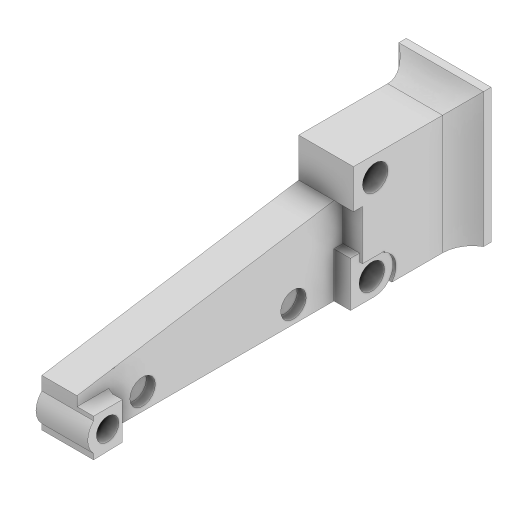
# Autodesk Inventor part: MotorAP
Saved by Autodesk Inventor 2023 (Build 270158030, 158C)
## iProperties
Created: 2022-08-10
Part Number: MotorAP
Material: Generic
Document SubType Name: Modeling
Designer: Ben
Density: 1 g/cm^3
Appearance: Default
Author: Ben
Autodesk Inventor part; units mm, degrees
sketch "Sketch1" plane through (0, 0, 0) normal (0, 0, 1) x (1, 0, 0)
  line L0 (0, 28.725) -> (20.5901, 28.725) projected
  line L1 (8.1353, 17.1738) -> (8.1353, 20.6738) projected
  line L2 (4.6353, 17.1738) -> (8.1353, 17.1738) projected
  line L3 (4.6353, 20.6738) -> (4.6353, 17.1738) projected
  line L4 (8.1353, 20.6738) -> (4.6353, 20.6738) projected
  line L5 (15.9861, 17.1738) -> (15.9861, 20.6738) projected
  line L6 (12.4861, 17.1738) -> (15.9861, 17.1738) projected
  line L7 (12.4861, 20.6738) -> (12.4861, 17.1738) projected
  line L8 (15.9861, 20.6738) -> (12.4861, 20.6738) projected
  circle A0 centre (14.2361, 18.9238) radius 1.75
  line L9 (0, 28.725) -> (0, 14.1337) projected
  line L10 (20.5901, 14.1337) -> (20.5901, 28.725) projected
  line L11 (0, 14.1337) -> (20.5901, 14.1337) projected
  constraints: 1 centre point, 1 tangent
sketch "Sketch2" plane through (0, 0, 0) normal (0, 0, 1) x (1, 0, 0)
  line L0 (13.8808, 28.6928) -> (10.5387, 28.6928)
  line L1 (10.5387, 28.6928) -> (10.5387, 20.7516)
  line L2 (10.5387, 20.7516) -> (13.8808, 20.7516)
  line L3 (14.1861, 26.5937) -> (14.1861, 28.0937)
  line L4 (14.1861, 20.7516) -> (13.8808, 20.7516)
  line L5 (13.8808, 28.6928) -> (14.1861, 28.6928)
  line L6 (14.5861, 22.7938) -> (13.9861, 22.7938)
  line L7 (14.1861, 26.0937) -> (14.5861, 26.0937)
  line L8 (14.1861, 26.0937) -> (15.1861, 26.0937)
  line L9 (15.1861, 26.0937) -> (15.1861, 22.7938)
  line L10 (15.1861, 22.7938) -> (14.1861, 22.7938)
  line L11 (14.1861, 28.6928) -> (14.1861, 26.0937)
  line L12 (14.1861, 22.7938) -> (14.1861, 20.7516)
  point P0 (0, 0)
  dimension "d2" = 1
  constraints: 26 end point, 4 perpendicular, 3 horizontal, 3 vertical, 2 parallel, 2 point on line, 6 other
  measures "d2" distance of L7.start L8.end
ref_plane "Work Plane1" through (12.8861, 20.2938, 3.59) normal (0, 0, -1) x (0, 1, 0)
extrude "Extrusion1" add sketch "Sketch2" along normal up to surface (3.59 mm away)
sketch "Sketch3" plane through (10.5387, 20.7516, 0) normal (-1, 0, 0) x (0, 0, 1)
  circle A0 centre (2.14, 6.5922) radius 0.75 projected
  circle A1 centre (2.17, 0.7922) radius 0.75 projected
  circle A2 centre (2.14, 6.5922) radius 0.85
  circle A3 centre (2.17, 0.7922) radius 0.85
  point P0 (0, -20.7516)
  dimension "d48" = 1.7
  dimension "d49" = 1.7
  constraints: 2 centre point, 2 coincident
  measures "d48" diameter of A2
  measures "d49" diameter of A3
extrude "Extrusion2" cut sketch "Sketch3" against normal up to next contours A0 | A1
ref_plane "Work Plane2" through (13.9861, 21.5438, 19.605) normal (-1, 0, 0) x (0, -1, 0)
sketch "Sketch5" plane through (13.9861, 21.5438, 19.605) normal (-1, 0, 0) x (0, -1, 0)
  line L0 (-4.5499, -16.015) -> (-7.149, -16.015) projected
  line L1 (-7.149, -16.015) -> (0.7922, -16.015) projected
  line L2 (0.7922, -16.015) -> (-1.25, -16.015) projected
  line L3 (-1.25, -16.015) -> (-4.5499, -16.015) projected
  circle A0 centre (0, 0.165) radius 0.75 projected
  line L4 (-4.5499, -16.015) -> (-7.149, -16.015) projected
  line L5 (1.3262, 1.5964) -> (-7.149, 1.5964)
  line L6 (-7.149, 1.5964) -> (-7.149, -16.015)
  line L7 (-7.149, -16.015) -> (1.3262, -16.015)
  line L8 (-4.5499, -19.605) -> (-4.5499, -16.015) projected
  line L9 (-1.7621, 1.5964) -> (-4.5499, -16.015)
  line L10 (0.7922, -19.605) -> (0.7922, -16.015) projected
  line L11 (0.7922, -19.605) -> (0.7922, -16.015) projected
  line L12 (0.7922, -16.015) -> (-1.25, -16.015) projected
  line L13 (0.7922, -16.015) -> (1.3262, 1.5964)
  circle A1 centre (0, 0.165) radius 0.85
  point P0 (21.5438, -19.605)
  dimension "d47" = 1.7
  constraints: 10 end point, 1 centre point, 1 coincident, 1 horizontal, 1 parallel, 1 perpendicular, 1 point on line
  measures "d47" diameter of A1
extrude "Extrusion3" add sketch "Sketch5" along normal up to surface (3.4474 mm away) contours L9 L5 L13 L1
sketch "Sketch6" plane through (13.9861, 21.5438, 19.605) normal (1, 0, 0) x (0, 0, -1)
  line L0 (16.015, 4.5499) -> (16.015, 7.149) projected
  line L1 (16.015, -0.7922) -> (-1.5964, -1.3262) projected
  line L2 (16.015, 7.149) -> (-1.5964, 7.149)
  line L3 (-1.5964, 7.149) -> (-1.5964, -1.3262)
  line L4 (-1.5964, -1.3262) -> (16.015, -1.3262)
  line L5 (16.015, -1.3262) -> (16.015, 7.149)
  point P0 (19.605, -21.5438)
  constraints: 8 end point, 2 parallel, 1 horizontal, 1 perpendicular
ref_plane "Work Plane3" through (12.8861, 20.2938, 3.59) normal (-1, 0, 0) x (0, 0, 1)
extrude "Extrusion4" cut sketch "Sketch6" against normal up to surface (1.1 mm away) contours L5 L1 L3 L2 L0
sketch "Sketch7" plane through (12.8861, 20.7516, 3.59) normal (1, 0, 0) x (0, 0, -1)
  line L0 (-14.6, 7.4422) -> (-14.6, -0.4578) projected
  line L1 (-17.6114, 2.5543) -> (0, 5.3422) projected
  line L2 (-14.6, -0.4578) -> (-14.6, 3.031)
  circle A0 centre (-16.18, 0.7922) radius 0.75 projected
  line L3 (0, 0) -> (-17.6114, -0.5339) projected
  line L4 (-17.6114, -0.5339) -> (-17.6114, 2.5543) projected
  point P0 (3.59, -20.7516)
  point P1 (-14.6, -0.4426)
  constraints: 2 end point, 2 point on line
ref_plane "Work Plane4" through (13.9861, 20.2938, 18.19) normal (-1, 0, 0) x (0, 0, 1)
extrude "Extrusion5" add sketch "Sketch7" along normal up to surface (1.1 mm away)
sketch "Sketch8" plane through (13.9861, 20.3089, 18.19) normal (1, 0, 0) x (0, 0, -1)
  arc A0 (-1.58, 2.4849) -> (-1.58, -0.0151) centre (-1.58, 1.2349) ccw projected
  line L0 (0, 2.5649) -> (-6.5, 2.5649)
  line L1 (-3.0114, -0.0913) -> (0, 0) projected
  line L2 (-3.0114, 2.997) -> (-3.0114, -0.0913) projected
  line L3 (-1.58, 2.4849) -> (-1.58, 2.5649)
  line L4 (-1.58, -0.0151) -> (-1.58, -0.0479)
  circle A1 centre (-1.58, 1.2349) radius 1.325
  line L5 (-2.5138, 2.1749) -> (-2.5138, 2.5649)
  line L6 (-2.5138, 0.2949) -> (-2.5138, -0.0762)
  point P0 (18.19, -20.3089)
  point P1 (-3.0114, 2.5649)
  dimension "d42" = 2.65
  constraints: 10 end point, 6 point on line, 2 point on circle, 1 centre point, 1 coincident, 1 horizontal, 1 perpendicular, 1 vertical, 2 other
  measures "d42" diameter of A1
ref_plane "Work Plane5" through (14.5861, 20.2938, 17.09) normal (1, 0, 0) x (0, 1, 0)
extrude "Extrusion6" add sketch "Sketch8" along normal up to surface (0.6 mm away) contours A1 L6 L1 L2 L0 L5
sketch "Sketch9" plane through (14.1861, 20.7516, 0) normal (1, 0, 0) x (0, 0, -1)
  circle A0 centre (-2.14, 6.5922) radius 0.75 projected
  line L0 (-3.59, 5.3422) -> (-3.59, 7.9412) projected
  line L1 (0, 5.3422) -> (-3.59, 5.3422) projected
  line L2 (0, 5.3422) -> (0, 7.9412) projected
  line L3 (0, 7.9412) -> (-3.59, 7.9412) projected
  line L4 (-3.59, 2.0422) -> (-3.59, 5.3422) projected
  line L5 (0, 2.0422) -> (-3.59, 2.0422) projected
  line L6 (0, 2.0422) -> (0, 5.3422) projected
  line L7 (0, 5.3422) -> (-3.59, 5.3422) projected
  circle A1 centre (-2.17, 0.7922) radius 0.75 projected
  line L8 (-3.59, 0) -> (-3.59, 2.0422) projected
  line L9 (0, 0) -> (-3.59, 0) projected
  line L10 (0, 0) -> (0, 2.0422) projected
  line L11 (0, 2.0422) -> (-3.59, 2.0422) projected
  point P0 (0, -20.7516)
ref_plane "Work Plane6" through (13.9861, 20.2938, 0.75) normal (-1, 0, 0) x (0, 0, 1)
sketch "Sketch10" plane through (14.1861, 20.7516, 0) normal (1, 0, 0) x (0, 0, -1)
  circle A0 centre (-2.17, 0.7922) radius 0.75 projected
  line L0 (-3.59, 0) -> (-3.59, 2.0422) projected
  line L1 (0, 0) -> (-3.59, 0) projected
  line L2 (0, 0) -> (0, 2.0422) projected
  line L3 (0, 2.0422) -> (-3.59, 2.0422) projected
  point P0 (0, -20.7516)
ref_plane "Work Plane7" through (13.9861, 20.2938, 0.75) normal (-1, 0, 0) x (0, 0, 1)
extrude "Extrusion8" cut sketch "Sketch10" against normal up to surface (0.2 mm away)
sketch "Sketch11" plane through (10.5387, 20.2176, 21.2014) normal (0, 0, 1) x (1, 0, 0)
  circle A0 centre (4.4974, 4.8062) radius 2.2 projected
  circle A1 centre (4.4974, 4.8062) radius 2.5
  point P0 (-10.5387, -20.2176)
  dimension "d46" = 5
  constraints: 1 centre point, 1 coincident
  measures "d46" diameter of A1
ref_plane "Work Plane8" through (12.8861, 20.2938, 18.19) normal (0, 0, 1) x (1, 0, 0)
extrude "Extrusion9" cut sketch "Sketch11" against normal up to surface (3.0114 mm away) contours A0 | A1
sketch "Sketch12" plane through (12.8861, 20.7516, 3.59) normal (1, 0, 0) x (0, 0, -1)
  circle A0 centre (-12.75, 0.6922) radius 0.85
  circle A1 centre (-2.7, 0.6922) radius 0.85
  line L0 (-3.4464, 0) -> (-2.0459, 0)
  point P0 (3.59, -20.7516)
  point P1 (-3.1933, 0)
  point P2 (-2.2067, 0)
  dimension "d40" = 1.7
  dimension "d41" = 1.7
  constraints: 2 centre point, 2 end point, 1 horizontal
  measures "d40" diameter of A0
  measures "d41" diameter of A1
extrude "Extrusion10" cut sketch "Sketch12" against normal blind 0.6 contours A0 | A1 L0 picked at (-2.6162, 0.9299)
sketch "Sketch13" plane through (14.1861, 26.0937, 0) normal (1, 0, 0) x (0, 0, -1)
  arc A0 (-2.14, 0) -> (-3.0564, 2.1001) centre (-2.14, 1.25) ccw projected
  line L0 (-1.9353, 2.4831) -> (-1.9353, 2.5991)
  line L1 (0, 2.5991) -> (-3.59, 2.5991) projected
  line L2 (0, 0) -> (0, 2.5991)
  line L3 (-1.6782, 0.0884) -> (-1.6782, 0)
  arc A1 (-2.14, 0) -> (-3.0564, 2.1001) centre (-2.14, 1.25) ccw projected
  circle A2 centre (-2.14, 1.25) radius 1.25
  line L4 (0, 0) -> (-3.59, 0) projected
  line L5 (-1.6782, 0) -> (0, 0)
  point P0 (0, -26.0937)
  constraints: 8 end point, 3 vertical, 2 point on circle, 1 centre point, 1 coincident, 1 concentric, 1 horizontal, 1 point on line
extrude "Extrusion11" add sketch "Sketch13" along normal up to surface (1 mm away) contours A0 L0 L1 L2 L4 L3
sketch "Sketch16" plane through (13.9861, 20.7516, 3.59) normal (1, 0, 0) x (0, 0, -1)
  line L0 (3.59, 7.9412) -> (3.59, 0) projected
  line L1 (3.59, 2.0422) -> (0, 2.0422) projected
  line L2 (3.59, 0) -> (2.0582, 0)
  line L3 (2.0582, 0) -> (2.0582, 2.0422)
  line L4 (2.0582, 2.0422) -> (3.59, 2.0422)
  line L5 (3.59, 2.0422) -> (3.59, 0)
  arc A0 (1.59, -0.4578) -> (1.59, 2.0422) centre (1.59, 0.7922) ccw projected
  point P0 (3.59, -20.7516)
  point P1 (2.0582, 1.9512)
  point P2 (2.5569, 0)
  constraints: 8 end point, 2 parallel, 1 horizontal, 1 perpendicular, 1 point on line
extrude "Extrusion12" add sketch "Sketch16" along normal up to surface (1.2 mm away) contours L0 L2 A0 L3 L1
sketch "Sketch18" plane through (10.5387, 20.2176, 21.2014) normal (-1, 0, 0) x (0, 0, 1)
  arc A0 (-18.3114, 7.1261) -> (-18.3114, 7.1261) centre (-19.0614, 7.1261) ccw projected
  arc A1 (-18.2814, 1.3262) -> (-18.2814, 1.3262) centre (-19.0314, 1.3262) ccw projected
  circle A2 centre (-19.0614, 7.1261) radius 1.25
  circle A3 centre (-19.0314, 1.3262) radius 1.25
  line L0 (-17.6114, 8.4752) -> (-17.6114, 5.8761) projected
  line L1 (-17.6114, 8.4752) -> (-17.6114, 0.5362)
  line L2 (-20.1683, 0.5339) -> (-17.6114, 0.5339) projected
  line L3 (-17.6114, 0.5362) -> (-17.6114, 0.5339)
  line L4 (-20.6002, 0.5339) -> (-20.6002, 8.4752) projected
  line L5 (-17.6114, 8.4752) -> (-20.6002, 8.4752)
  line L6 (-20.6002, 8.4752) -> (-20.6002, 0.5339)
  line L7 (-20.6002, 0.5339) -> (-19.9983, 0.5339)
  line L8 (-20.6002, 0.5339) -> (-17.6114, 0.5339)
  point P0 (-21.2014, -20.2176)
  point P1 (-18.0645, 0.5339)
  dimension "d27" = 2.5
  constraints: 12 end point, 3 perpendicular, 2 coincident, 1 centre point, 1 collinear, 1 point on line, 1 vertical, 3 other
extrude "Extrusion14" cut sketch "Sketch18" along normal through all contours A0 | A1 | A2 | A3 L2 picked at (-17.9599, 1.4249)
sketch "Sketch19" plane through (15.1861, 22.7938, 3.59) normal (1, 0, 0) x (0, 0, -1)
  line L0 (1.9118, 3.2999) -> (0, 3.2999) projected
  line L1 (2.9889, -2.0422) -> (2.9889, 5.899) projected
  line L2 (1.0967, 3.2999) -> (2.9889, 3.2999)
  line L3 (2.9889, 3.2999) -> (2.9889, 5.899)
  line L4 (2.9889, 5.899) -> (1.0967, 5.899)
  line L5 (1.0967, 5.899) -> (1.0967, 3.2999)
  circle A0 centre (1.4413, 4.5476) radius 1.5803
  point P0 (3.59, -22.7938)
  point P1 (0.4713, 3.2999)
  point P2 (2.4113, 3.2999)
  constraints: 8 end point, 2 parallel, 1 centre point, 1 horizontal, 1 perpendicular, 1 point on line
ref_plane "Work Plane9" through (14.5861, 26.0937, 0.89) normal (1, 0, 0) x (0, 1, 0)
extrude "Extrusion15" cut sketch "Sketch19" against normal up to surface (0.6 mm away) contours L2 A0 L0 | L0 L5 L4 A0 L1 L2 | A0 L1 L2 | L4 L1 A0
sketch "Sketch20" plane through (15.1861, 22.7938, 3.59) normal (1, 0, 0) x (0, 0, -1)
  line L0 (2.0582, 0) -> (0, 0) projected
  line L1 (2.9889, -2.0422) -> (3.59, -2.0422) projected
  line L2 (2.0582, 0) -> (2.9889, 0)
  line L3 (2.9889, 0) -> (2.9889, -2.0422)
  line L4 (2.9889, -2.0422) -> (2.0582, -2.0422)
  line L5 (2.0582, -2.0422) -> (2.0582, 0)
  circle A0 centre (1.4197, -1.2443) radius 1.5589
  point P0 (3.59, -22.7938)
  point P1 (2.3588, 0)
  point P2 (0.4807, 0)
  constraints: 8 end point, 2 parallel, 1 centre point, 1 horizontal, 1 perpendicular
ref_plane "Work Plane10" through (14.5861, 20.2938, 0.75) normal (1, 0, 0) x (0, 1, 0)
extrude "Extrusion16" cut sketch "Sketch20" against normal up to surface (0.6 mm away) contours L0 A0 L2 | L2 A0 L4 L5 | L2 L3 L4 A0
sketch "Sketch21" plane through (15.1861, 22.7938, 3.59) normal (1, 0, 0) x (0, 0, -1)
  line L0 (0.4713, 3.2999) -> (1.9118, 3.2999) projected
  arc A0 (0.4713, 3.2999) -> (2.4113, 3.2999) centre (1.4413, 4.5476) ccw projected
  line L1 (2.9889, 3.2999) -> (2.4113, 3.2999) projected
  line L2 (2.9889, 5.899) -> (2.9889, 3.2999) projected
  line L3 (1.6547, 5.899) -> (2.9889, 5.899) projected
  line L4 (1.6547, 5.783) -> (1.6547, 5.899) projected
  arc A1 (1.9118, 3.3884) -> (1.6547, 5.783) centre (1.45, 4.5499) ccw projected
  line L5 (1.9118, 3.2999) -> (1.9118, 3.3884) projected
  arc A2 (2.3588, 0) -> (0.4807, 0) centre (1.4197, -1.2443) ccw projected
  line L6 (2.3588, 0) -> (2.9889, 0) projected
  line L7 (2.9889, 3.2999) -> (2.4113, 3.2999) projected
  arc A3 (0.4713, 3.2999) -> (2.4113, 3.2999) centre (1.4413, 4.5476) ccw projected
  line L8 (0.4713, 3.2999) -> (0, 3.2999) projected
  line L9 (0, 0) -> (0, 3.2999) projected
  line L10 (0.4807, 0) -> (0, 0) projected
  line L11 (0, 0) -> (0, 3.2999) projected
  line L12 (0.4713, 3.2999) -> (1.9118, 3.2999) projected
  line L13 (0, 0.5118) -> (0.6, 0.5118)
  line L14 (0.6, 0.5118) -> (0.6, 3.2999)
  line L15 (0.6, 3.2999) -> (0, 3.2999)
  line L16 (0, 3.2999) -> (0, 0.5118)
  line L17 (2.9889, 0) -> (2.9889, -2.0422) projected
  line L18 (3.59, -2.0422) -> (2.9889, -2.0422) projected
  line L19 (3.59, 5.899) -> (3.59, -2.0422) projected
  line L20 (2.9889, 5.899) -> (3.59, 5.899) projected
  line L21 (2.9889, 5.899) -> (2.9889, 3.2999) projected
  point P0 (3.59, -22.7938)
  point P1 (0.6, 3.2098)
  point P2 (0.4713, 3.2999)
  dimension "d34" = 0.6
  constraints: 8 end point, 2 parallel, 2 point on line, 1 horizontal, 1 perpendicular
  measures "d34" distance of L15.end L14.end
extrude "Extrusion17" cut sketch "Sketch21" against normal up to surface (2.3 mm away) contours L0 L14 A0 | A0 L14 L13 L9 L8
sketch "Sketch22" plane through (13.9861, 20.7516, 3.59) normal (1, 0, 0) x (0, 0, -1)
  line L0 (2.0582, 1.9512) -> (2.0582, 2.0422) projected
  line L1 (2.0582, 2.0422) -> (0, 2.0422) projected
  line L2 (0, 0) -> (0, 2.0422) projected
  line L3 (2.5569, 0) -> (0, 0) projected
  arc A0 (2.5569, 0) -> (2.0582, 1.9512) centre (1.59, 0.7922) ccw projected
  circle A1 centre (1.42, 0.7922) radius 0.75 projected
  line L4 (0, 0) -> (0, 2.0422) projected
  line L5 (2.5569, 0) -> (0, 0) projected
  circle A2 centre (1.42, 0.7922) radius 1.1389
  arc A3 (1.7542, -0.2966) -> (2.5569, 0) centre (1.4857, 1.6649) ccw
  point P0 (3.59, -20.7516)
  point P1 (0.6018, 0)
  constraints: 2 point on circle, 1 centre point, 1 coincident, 3 other
ref_plane "Work Plane11" through (12.8861, 20.2938, 3.59) normal (-1, 0, 0) x (0, 0, 1)
extrude "Extrusion18" cut sketch "Sketch22" against normal up to surface (1.1 mm away) contours A0 L3 A2 L2 L1 L0 | A3 A2 L3 | A2 L3 | L3 A2 | A1
sketch "Sketch23" plane through (13.9861, 21.5438, 19.77) normal (1, 0, 0) x (0, 0, -1)
  line L0 (-0.9338, 1.2112) -> (-0.9338, 0.94) projected
  arc A0 (-0.9338, 0.94) -> (-0.9338, -0.94) centre (0, 0) ccw projected
  line L1 (-0.9338, -0.94) -> (-0.9338, -1.3111) projected
  line L2 (-0.9338, -1.3111) -> (1.58, -1.2349) projected
  line L3 (1.58, -1.2349) -> (1.58, 1.2112) projected
  line L4 (-0.9338, -1.3111) -> (1.58, -1.2349) projected
  line L5 (0.98, -1.2531) -> (0.98, 2.1438)
  line L6 (1.58, 1.2112) -> (-0.9338, 1.2112) projected
  line L7 (1.58, 1.2112) -> (-0.9338, 1.2112) projected
  line L8 (1.58, 2.2043) -> (1.58, 1.2112) projected
  line L9 (-1.4314, 1.7621) -> (1.58, 2.2388) projected
  line L10 (-1.4314, 1.0208) -> (-1.4314, 1.7621) projected
  line L11 (1.58, 2.2043) -> (1.58, 2.2388) projected
  line L12 (-0.9338, 1.0208) -> (-1.4314, 1.0208) projected
  line L13 (-0.9338, 1.2112) -> (-0.9338, 1.0208) projected
  point P0 (19.77, -21.5438)
  point P1 (0.98, -1.2531)
  point P2 (0.98, 1.2112)
  point P3 (0.98, 1.2112)
  constraints: 2 end point, 2 point on line, 1 vertical
ref_plane "Work Plane12" through (12.8861, 20.2938, 3.59) normal (-1, 0, 0) x (0, 0, 1)
extrude "Extrusion19" cut sketch "Sketch23" against normal up to surface (1.1 mm away) contours L0 L12 L10 L9 L5 L6 | L6 L3 L2 L5 | L5 L9 L11 L8 L6
sketch "Sketch24" plane through (10.5387, 20.2176, 21.2014) normal (-1, 0, 0) x (0, 0, 1)
  circle A0 centre (-19.0614, 7.1261) radius 0.75 projected
  circle A1 centre (-19.0314, 1.3262) radius 0.75 projected
  circle A2 centre (-19.0614, 7.1261) radius 0.85
  circle A3 centre (-19.0314, 1.3262) radius 0.85
  point P0 (-21.2014, -20.2176)
  dimension "d50" = 1.7
  dimension "d51" = 1.7
  constraints: 2 centre point, 2 coincident
  measures "d50" diameter of A2
  measures "d51" diameter of A3
extrude "Extrusion20" cut sketch "Sketch24" against normal up to next contours A0 | A1 | A2 | A3
sketch "Sketch25" plane through (14.5861, 21.5438, 19.77) normal (1, 0, 0) x (0, 0, -1)
  line L0 (-0.9338, 1.0208) -> (-1.4314, 1.0208) projected
  line L1 (-1.4314, -1.3262) -> (-1.4314, 1.0208) projected
  line L2 (-0.9338, -1.3111) -> (-1.4314, -1.3262) projected
  line L3 (-0.9338, -0.94) -> (-0.9338, -1.3111) projected
  arc A0 (-0.9338, 0.94) -> (-0.9338, -0.94) centre (0, 0) ccw projected
  line L4 (-0.9338, 1.0208) -> (-0.9338, 0.94) projected
  line L5 (-0.9338, 1.0208) -> (-1.4314, 1.0208) projected
  line L6 (-1.4314, 1.0208) -> (-0.9338, 1.0208)
  line L7 (-0.9338, 1.0208) -> (-0.9338, 2.2284)
  line L8 (-0.9338, 2.2284) -> (-1.4314, 2.2284)
  line L9 (-1.4314, 2.2284) -> (-1.4314, 1.0208)
  point P0 (19.77, -21.5438)
  constraints: 8 end point, 2 parallel, 1 horizontal, 1 perpendicular
extrude "Extrusion21" cut sketch "Sketch25" against normal up to next
sketch "Sketch26" plane through (10.5387, 20.7516, 3.59) normal (0, -0.9995407, -0.0303043) x (1, 0, 0)
  line L0 (3.4474, 17.1217) -> (0, 17.1217) projected
  line L1 (0, 17.1217) -> (0, 0) projected
  line L2 (0, 0) -> (2.3474, 0) projected
  line L3 (2.3474, 0) -> (2.3474, 15.207) projected
  line L4 (2.3474, 15.207) -> (3.4474, 15.207) projected
  line L5 (3.4474, 17.1217) -> (3.4474, 15.207) projected
  line L6 (2.3474, 0) -> (2.3474, 15.207) projected
  line L7 (2.3474, 14.9376) -> (2.9742, 15.207)
  line L8 (2.3474, 15.207) -> (3.4474, 15.207) projected
  point P0 (-10.5387, -2.9595)
  point P1 (2.3474, 14.9376)
  point P2 (2.9742, 15.207)
  constraints: 2 end point, 2 point on line
extrude "Extrusion22" add sketch "Sketch26" against normal up to surface contours L7 L3 L4 surface through (13.9861, 22.755, 18.79) normal (0, -1, 0)
sketch "Sketch27" plane through (15.1861, 26.0937, 1.1787) normal (1, 0, 0) x (0, 0, -1)
  line L0 (-1.9306, -3.2999) -> (-2.4113, -3.2999) projected
  line L1 (-1.8113, -0.0901) -> (-1.8113, -2.7881) projected
  line L2 (-2.4113, -3.2999) -> (-1.8113, -3.2999)
  line L3 (-1.8113, -3.2999) -> (-1.8113, -2.7881)
  line L4 (-1.8113, -2.7881) -> (-2.4113, -2.7881)
  line L5 (-2.4113, -2.7881) -> (-2.4113, -3.2999)
  point P0 (1.1787, -26.0937)
  constraints: 8 end point, 2 parallel, 1 horizontal, 1 perpendicular
extrude "Extrusion23" cut sketch "Sketch27" against normal up to surface (1.2 mm away)
sketch "Sketch29" plane through (14.5861, 26.0937, 0.6011) normal (1, 0, 0) x (0, 0, -1)
  line L0 (-2.3889, 0) -> (-2.3889, -0.0901) projected
  arc A0 (-2.3889, -0.0901) -> (-0.5776, 0) centre (-1.5476, 1.2477) ccw projected
  line L1 (0, 0) -> (-0.5776, 0) projected
  line L2 (0, 2.5991) -> (0, 0) projected
  line L3 (-1.3342, 2.5991) -> (0, 2.5991) projected
  line L4 (-1.3342, 2.4831) -> (-1.3342, 2.5991) projected
  arc A1 (-1.0771, 0.0884) -> (-1.3342, 2.4831) centre (-1.5389, 1.25) ccw projected
  line L5 (-1.0771, 0) -> (-1.0771, 0.0884) projected
  line L6 (-2.3889, 0) -> (-1.0771, 0) projected
  point P0 (0.6011, -26.0937)
extrude "Extrusion25" cut sketch "Sketch29" against normal up to surface (0.4 mm away)
sketch "Sketch30" plane through (15.1861, 26.0937, 1.1787) normal (1, 0, 0) x (0, 0, -1)
  line L0 (-1.8113, -0.0901) -> (-1.8113, -3.2183) projected
  arc A0 (-0.0525, -3.2999) -> (-1.8113, -3.2183) centre (-0.9916, -4.5442) ccw projected
  line L1 (-0.0525, -3.2999) -> (0.5776, -3.2999) projected
  line L2 (0.5776, 0) -> (0, 0) projected
  arc A1 (-1.8113, -0.0901) -> (0, 0) centre (-0.97, 1.2477) ccw projected
  line L3 (-1.8113, -0.0901) -> (-1.8113, -3.2183) projected
  line L4 (0.5776, -5.3422) -> (0.5776, -3.2999) projected
  line L5 (-1.8113, 0.6335) -> (0.5776, 0.6335)
  line L6 (0.5776, 0.6335) -> (0.5776, -3.2999)
  line L7 (0.5776, -3.2999) -> (-1.8113, -3.2999)
  line L8 (-1.8113, -3.2999) -> (-1.8113, 0.6335)
  line L9 (0.5776, -3.2999) -> (0.5776, -5.3422) projected
  line L10 (1.1787, -5.3422) -> (0.5776, -5.3422) projected
  line L11 (1.1787, 2.5991) -> (1.1787, -5.3422) projected
  line L12 (0.5776, 2.5991) -> (1.1787, 2.5991) projected
  line L13 (0.5776, 2.5991) -> (0.5776, 0) projected
  point P0 (1.1787, -26.0937)
  constraints: 8 end point, 2 parallel, 1 horizontal, 1 perpendicular, 1 point on line
extrude "Extrusion26" cut sketch "Sketch30" against normal up to surface (1 mm away) contours A1 L2 L6 L1 A0 L0 | L6 L13 L12 L11 L10 L4
sketch "Sketch32" plane through (10.5387, 26.0937, 3.59) normal (-1, 0, 0) x (0, 0, 1)
  line L0 (17.1138, -3.6099) -> (17.1138, -2.7091) projected
  line L1 (0, 0) -> (17.1138, -2.7091) projected
  line L2 (0, 2.5991) -> (0, 0) projected
  line L3 (-3.59, 2.5991) -> (0, 2.5991) projected
  line L4 (-3.59, -5.3422) -> (-1.728, -5.3422) projected
  arc A0 (-1.112, -5.3422) -> (-1.728, -5.3422) centre (-1.42, -4.5499) ccw projected
  line L5 (-1.112, -5.3422) -> (0, -5.3422) projected
  line L6 (17.1138, -5.861) -> (0, -5.3422) projected
  line L7 (17.1138, -5.861) -> (17.1138, -5.4899) projected
  arc A1 (17.1138, -5.4899) -> (17.1138, -3.6099) centre (16.18, -4.5499) ccw projected
  circle A2 centre (16.18, -4.5499) radius 0.85 projected
  circle A3 centre (-1.45, 1.25) radius 0.85 projected
  line L8 (14.6, -5.7999) -> (0, -5.7999) projected
  line L9 (1.41, -5.7999) -> (-8.59, -5.7999) projected
  line L10 (-3.59, 2.6313) -> (-3.59, -26.0937) projected
  line L11 (-3.59, -5.3422) -> (-2.3869, -5.3422) projected
  line L12 (-1.112, -5.3422) -> (-1.728, -5.3422)
  line L13 (-3.59, 2.5991) -> (-3.59, -5.3422) projected
  line L14 (-3.59, -5.3422) -> (-3.59, -5.7999)
  line L15 (0, -5.3422) -> (14.9307, -5.7948) projected
  line L16 (-3.59, -5.7999) -> (14.9307, -5.7948)
  arc A4 (-1.112, -5.3422) -> (-1.728, -5.3422) centre (-1.42, -4.5499) ccw projected
  line L17 (-1.728, -5.3422) -> (-3.59, -5.3422)
  line L18 (-1.112, -5.3422) -> (0, -5.3422) projected
  line L19 (-1.112, -5.3422) -> (1.3559, -5.2481)
  line L20 (1.3559, -5.2481) -> (6.0099, -5.4899)
  line L21 (6.0099, -5.4899) -> (14.9307, -5.4899)
  line L22 (14.9307, -5.4899) -> (14.9307, -5.7948)
  circle A5 centre (-1.42, -4.5499) radius 0.85
  line L23 (-3.59, 2.5991) -> (-3.59, -5.3422) projected
  constraints: 16 end point, 1 coincident, 1 midpoint, 1 perpendicular, 1 point on line, 3 other
extrude "Extrusion28" add sketch "Sketch32" against normal up to surface (2.3474 mm away) contours L16 L8 L9 L10 L4 A5 L5 L6 | L6 L5 L19 L20 L21 L22
sketch "Sketch33" plane through (12.8861, 23.3056, 2.99) normal (1, 0, 0) x (0, 0, -1)
  line L0 (-3.7658, -2.554) -> (-3.7933, -2.554) projected
  arc A0 (-2.7394, -2.5007) -> (-3.7933, -2.554) centre (-3.3, -1.8618) ccw projected
  line L1 (-2.7394, -2.5007) -> (-3.7658, -2.554) projected
  arc A1 (-13.2201, -2.7018) -> (-13.4799, -2.7018) centre (-13.35, -1.8618) ccw projected
  line L2 (-13.2201, -2.7018) -> (-13.4799, -2.7018) projected
  line L3 (-15.5307, -3.0067) -> (2.99, -3.0118) projected
  line L4 (2.99, -3.0118) -> (2.99, -2.554) projected
  line L5 (1.9569, -2.554) -> (2.99, -2.554) projected
  circle A2 centre (0.82, -1.7618) radius 0.85 projected
  line L6 (-0.6, -0.5118) -> (-0.6, 0) projected
  line L7 (-0.6, 0) -> (0, 0) projected
  line L8 (0, 0) -> (0, 2.7881) projected
  line L9 (0, 2.7881) -> (-0.6, 2.7881) projected
  line L10 (-15.2, 0.477) -> (-0.6, 2.7881) projected
  line L11 (-15.2, 0.477) -> (-15.2, 0.4425) projected
  line L12 (-15.418, 0.4425) -> (-15.2, 0.4425) projected
  line L13 (-17.7138, 0.079) -> (-15.418, 0.4425) projected
  line L14 (-17.7138, 0.079) -> (-17.7138, -0.5506) projected
  line L15 (-17.7138, -0.5506) -> (-15.6052, -0.5506) projected
  line L16 (-15.6052, -0.5506) -> (-15.5307, -3.0067) projected
  circle A3 centre (-3.3, -1.8618) radius 0.85
  circle A4 centre (-13.35, -1.8618) radius 0.85
  arc A5 (1.9569, -2.554) -> (1.4582, -0.6028) centre (0.99, -1.7618) ccw projected
  line L17 (1.4582, -0.6028) -> (1.4582, -0.5118) projected
  line L18 (1.4582, -0.5118) -> (-0.6, -0.5118) projected
  point P0 (2.99, -23.3056)
  point P1 (-2.7394, -2.5007)
  constraints: 2 centre point, 2 coincident, 1 concentric
extrude "Extrusion29" cut sketch "Sketch33" against normal up to surface (0.6 mm away) contours L1 A3 L0 | L0 A0 L1 | L2 A1 | A4 L2
sketch "Sketch35" plane through (14.5861, 22.7028, 1.5318) normal (1, 0, 0) x (0, 0, -1)
  line L0 (-1.4582, 0.1727) -> (-1.4582, 0.091) projected
  line L1 (0, 0.091) -> (-1.4582, 0.091) projected
  line L2 (0, 0) -> (0, 0.091) projected
  arc A0 (0.4987, -1.9512) -> (0, 0) centre (-0.4682, -1.159) ccw projected
  line L3 (0.9307, -1.9512) -> (0.4987, -1.9512) projected
  line L4 (0.9307, 0.091) -> (0.9307, -1.9512) projected
  line L5 (0.3005, 0.091) -> (0.9307, 0.091) projected
  arc A1 (0.3005, 0.091) -> (-1.4582, 0.1727) centre (-0.6385, -1.1533) ccw projected
  point P0 (1.5318, -22.7028)
extrude "Extrusion31" cut sketch "Sketch35" against normal up to surface (0.4 mm away)
sketch "Sketch37" plane through (12.8861, 22.7938, 3.59) normal (1, 0, 0) x (0, 0, -1)
  arc A0 (1.59, -2.5) -> (1.59, 0) centre (1.59, -1.25) ccw projected
  line L0 (1.59, 0) -> (0, 0) projected
  line L1 (0, 0) -> (0, -1.8) projected
  line L2 (0, -1.8) -> (-1.5, -1.8) projected
  line L3 (-1.5, -1.8) -> (-1.5, -2.5) projected
  line L4 (-1.5, -2.5) -> (1.59, -2.5) projected
  circle A1 centre (1.42, -1.25) radius 0.75 projected
  line L5 (0, -1.8) -> (0, -2.499)
  line L6 (3.59, -2.5) -> (-14.9307, -2.4949) projected
  circle A2 centre (1.42, -1.25) radius 0.85 projected
  point P0 (3.59, -22.7938)
  point P1 (1.6267, -2.4995)
  constraints: 2 end point, 1 perpendicular, 1 point on line
ref_plane "Work Plane13" through (13.9861, 20.2938, 0.75) normal (-1, 0, 0) x (0, 0, 1)
extrude "Extrusion32" add sketch "Sketch37" along normal up to surface (1.1 mm away) contours L4 L5 L1 L0 A0
sketch "Sketch38" plane through (0, 0, 0) normal (0, 0, -1) x (-1, 0, 0)
  line L0 (-14.1861, 28.6928) -> (-14.1861, 20.7516) projected
  line L1 (-12.8861, 20.7516) -> (-14.1861, 20.7516) projected
  line L2 (-12.8861, 20.2938) -> (-12.8861, 20.7516) projected
  line L3 (-10.5387, 20.2938) -> (-12.8861, 20.2938) projected
  line L4 (-10.5387, 28.6928) -> (-10.5387, 20.2938) projected
  line L5 (-14.1861, 28.6928) -> (-10.5387, 28.6928) projected
  point P0 (0, 0)
extrude "Extrusion33" add sketch "Sketch38" along normal blind 4.575
sketch "Sketch39" plane through (12.8861, 22.7028, 1.5318) normal (1, 0, 0) x (0, 0, -1)
  arc A0 (0, 0) -> (-0.4682, 0.091) centre (-0.4682, -1.159) ccw projected
  line L0 (0, 0) -> (0, 0.091) projected
  line L1 (0, 0.091) -> (-0.4682, 0.091) projected
  point P0 (1.5318, -22.7028)
extrude "Extrusion34" add sketch "Sketch39" along normal blind 1.1
sketch "Sketch40" plane through (0, 0, -4.575) normal (0, 0, -1) x (-1, 0, 0)
  line L0 (-14.1861, 28.6928) -> (-14.1861, 20.7516)
  line L1 (-12.8861, 20.7516) -> (-12.8861, 20.2938)
  line L2 (-10.5387, 20.7516) -> (-10.5387, 28.6928)
  line L3 (-10.5387, 28.6928) -> (-14.1861, 28.6928)
  line L4 (-15.1861, 20.7516) -> (-15.1861, 29.6928)
  line L5 (-15.1861, 29.6928) -> (-9.5387, 29.6928)
  line L6 (-9.5387, 29.6928) -> (-9.5387, 20.7516)
  line L7 (-15.1861, 20.7516) -> (-9.5387, 20.7516)
  point P0 (0, 0)
  constraints: 16 end point, 1 perpendicular, 1 point on line
extrude "Extrusion35" add sketch "Sketch40" against normal blind 0.5 contours L0 L7 L4 L5 L6 L2 L3
fillet "Fillet2" radius 2 3 edges at (14.1861, 24.7222, -4.075) (12.3624, 28.6928, -4.075) (10.5387, 24.7222, -4.075)
body "Solid1"
